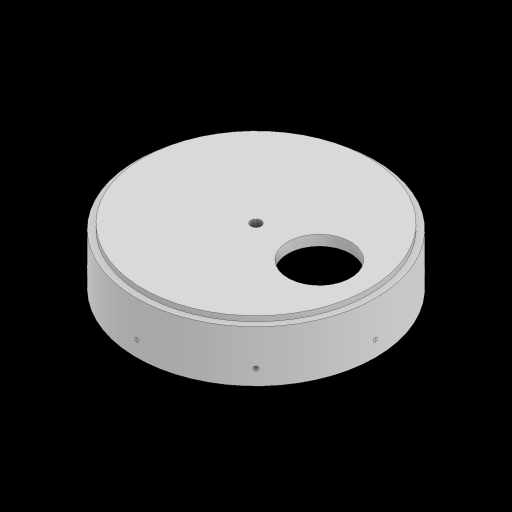
# Autodesk Inventor part: SC-1-01-Housing lid
Saved by Autodesk Inventor 2023 (Build 270158000, 158)
## iProperties
Created: 2023-12-31
Part Number: SC-1-01-Housing lid
Material: Generic
Document SubType Name: Modeling
Designer: annah
Density: 1 g/cm^3
Appearance: Default
Author: annah
Autodesk Inventor part; units mm, degrees
ref_plane "YZ Plane" through (0, 0, 0) normal (1, 0, 0) x (0, 1, 0)
ref_plane "XZ Plane" through (0, 0, 0) normal (0, 1, 0) x (-1, 0, 0)
sketch "Sketch1" plane through (0, 0, 0) normal (0, 1, 0) x (-1, 0, 0)
  circle A0 centre (0, 0) radius 65.0875
  circle A1 centre (0, -39.0525) radius 19.3675
  circle A2 centre (39.0525, 0) radius 19.3675
  circle A3 centre (0, 39.0525) radius 19.3675
  circle A4 centre (-39.0525, 0) radius 19.3675
  circle A5 centre (0, 0) radius 3.175
  circle A6 centre (0, 0) radius 69.85
  dimension "d2" = 130.175
  dimension "d3" = 38.735
  dimension "d4" = 39.0525
  dimension "d5" = 360
  dimension "d6" = 6.35
  dimension "d7" = 139.7
  constraints: 7 centre point, 2 coincident, 9 other
  measures "d2" diameter of A0
  measures "d3" diameter of A1
  measures "d4" distance of point (0, 0) A1.centre
  measures "d6" diameter of A5
  measures "d7" diameter of A6
extrude "Extrusion1" add sketch "Sketch1" along normal blind 19.05 contours A0 | A1 | A2 | A3 | A6
sketch "Sketch2" plane through (0, 0, 0) normal (0, -1, 0) x (1, 0, 0)
  circle A0 centre (0, 0) radius 3.175 projected
  circle A1 centre (0, 0) radius 67.4688
  dimension "d10" = 134.9375
  constraints: 1 centre point, 1 coincident
  measures "d10" diameter of A1
extrude "Extrusion2" cut sketch "Sketch2" against normal blind 12.7 contours A0 | A1
sketch "Sketch3" plane through (0, 0, 0) normal (0, -1, 0) x (1, 0, 0)
  circle A0 centre (0, 0) radius 3.175 projected
  circle A1 centre (0, 0) radius 73.66
  circle A2 centre (0, 0) radius 67.4688
  circle A3 centre (0, 0) radius 69.85
  dimension "d13" = 147.32
  constraints: 3 centre point, 3 coincident
  measures "d13" diameter of A1
extrude "Extrusion3" add sketch "Sketch3" along normal mid plane 31.75 contours A1
ref_plane "Work Plane1" through (0, 0, 73.66) normal (0, 0, 1) x (1, 0, 0)
sketch "Sketch4" plane through (0, 0, 73.66) normal (0, 0, 1) x (1, 0, 0)
  circle A0 centre (0, -6.35) radius 1.27
  line L0 (73.66, 15.875) -> (-73.66, 15.875) projected
  line L1 (-73.66, -15.875) -> (73.66, -15.875) projected
  point P0 (0, 0)
  dimension "d17" = 2.54
  dimension "d30" = 9.525
  constraints: 1 centre point
  measures "d17" diameter of A0
  measures "d30" distance from line of L1 A0.centre
extrude "Extrusion4" cut sketch "Sketch4" against normal up to surface round surface about axis through (0, 0, 0) along (0, -1, 0) radius 69.85 far side no
pattern_circular "Circular Pattern1" count 8 over 360 about axis through (0, -10, 0) along (0, 1, 0) of "Extrusion4"
extrude "Extrusion5" add sketch "Sketch4" against normal up to surface round surface about axis through (0, 0, 0) along (0, -1, 0) radius 73.66 far side no
pattern_circular "Circular Pattern2" count 4 over 360 about axis through (0, -10, 0) along (0, 1, 0) of "Extrusion5"
equation "\"d4\" = 0.3 * d2"
body "Solid1"
